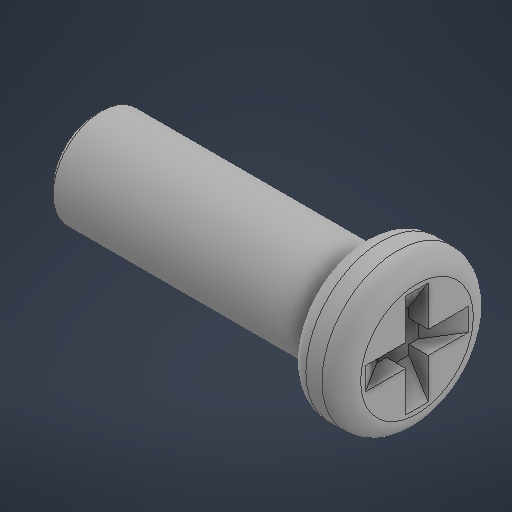
# Autodesk Inventor part: screw
Saved by Autodesk Inventor 2025.2 (Build 292293000, 293)
## iProperties
Created: 2025-11-04
Part Number: screw
Material: Generic
Document SubType Name: Modeling
Designer: micyg
Density: 1 g/cm^3
Appearance: Default
Author: micyg
Autodesk Inventor part; units mm, degrees
ref_plane "YZ Plane" through (0, 0, 0) normal (1, 0, 0) x (0, 1, 0)
ref_plane "XZ Plane" through (0, 0, 0) normal (0, 1, 0) x (-1, 0, 0)
ref_plane "XY Plane" through (0, 0, 0) normal (0, 0, 1) x (1, 0, 0)
sketch "Sketch1" plane through (0, 0, 0) normal (0, 1, 0) x (-1, 0, 0)
  line L0 (0, 0) -> (1.7, 0)
  line L1 (1.7, 0) -> (1.7, -1.75)
  line L2 (1.1, -2.35) -> (0.6, -2.35)
  line L3 (0, -1.75) -> (0, 0)
  line L4 (1.7, -1.5) -> (10, -1.5)
  line L5 (10, -1.5) -> (10, 0)
  line L6 (10, 0) -> (1.7, 0)
  line L7 (1.7, 0) -> (1.7, -1.5)
  line L8 (1.7, 0) -> (1.7, 2.35)
  line L9 (1.7, 2.35) -> (0, 2.35)
  line L10 (0, 2.35) -> (0, 0)
  line L11 (1.7, 1.5) -> (10, 1.5)
  line L12 (10, 1.5) -> (10, 0)
  arc A0 (1.1, -2.35) -> (1.7, -1.75) centre (1.1, -1.75) ccw
  arc A1 (0, -1.75) -> (0.6, -2.35) centre (0.6, -1.75) ccw
  point P0 (1.7, -2.35)
  point P1 (0, -2.35)
  dimension "d1" = 3
  dimension "d2" = 4.7
  dimension "d3" = 1.7
  dimension "d4" = 10
  dimension "d6" = 0.6
  dimension "d7" = 0.6
  constraints: 26 end point, 6 point on line, 4 parallel, 4 point on circle, 4 symmetric about line, 4 tangent, 2 centre point, 2 horizontal, 2 perpendicular, 1 other
  measures "d1" distance between parallel lines of L11 L4
  measures "d2" distance between parallel lines of L9 L2
  measures "d3" distance between parallel lines of L3 L1
  measures "d4" distance between parallel lines of L5 L3
  measures "d6" radius of A0
  measures "d7" radius of A1
revolve "Revolution1" add sketch "Sketch1" angle 360 about axis through (-10, 0, 0) along (1, 0, 0) contours L0 L1 A0 L2 A1 L3 | L6 L5 L4 L1
chamfer "Chamfer1" distance 0.2 angle 45 1 edges at (-10, 0, 1.5)
sketch "Sketch3" plane through (0, 0, 0) normal (0, 1, 0) x (-1, 0, 0)
  line L0 (0.6, 2.35) -> (0.6, -2.35) construction
  line L1 (0, 1.75) -> (0, -1.75) projected
  line L2 (0, -1.6) -> (1, 0)
  line L3 (1, 0) -> (0, 0)
  line L4 (1, 0) -> (0, 1.6)
  line L5 (0.6, -0.64) -> (0.6, 0.64)
  dimension "d11" = 3.2
  dimension "d12" = 1
  dimension "d18" = 0.6
  constraints: 8 end point, 4 point on line, 1 horizontal, 1 parallel, 1 other
  measures "d11" distance of L4.end L2.start
  measures "d12" distance of L2.end L3.end
  measures "d18" distance between parallel lines of L1 L5
extrude "Extrusion1" cut sketch "Sketch3" along normal mid plane 0.7 contours L4 L5 L3 L1 | L3 L5 L2 L1
pattern_circular "Circular Pattern1" count 2 over 90 about axis through (-0.85, 0, 0) along (1, 0, 0) of "Extrusion1"
equation "\"d6\" = d7"
body "Solid1"
